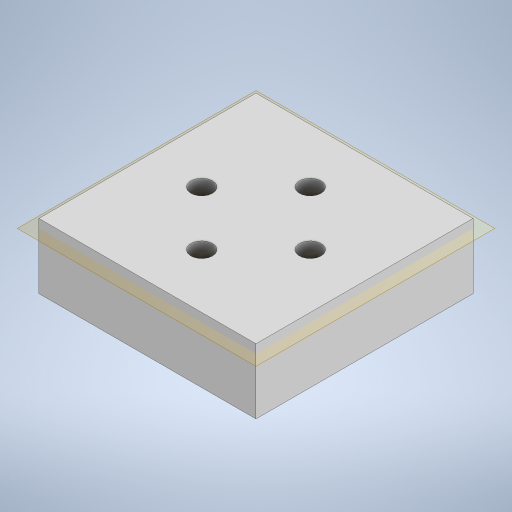
# Autodesk Inventor part: TestBauteil
Saved by Autodesk Inventor 2024.1 (Build 281209000, 209)
## iProperties
Created: 2023-11-30
Part Number: TestBauteil
Material: Generisch
Document SubType Name: Modeling
Designer: tobia
Density: 1 g/cm^3
Appearance: Vorgabe
Author: tobia
Autodesk Inventor part; units mm, degrees
ref_plane "YZ Plane" through (0, 0, 0) normal (1, 0, 0) x (0, 1, 0)
ref_plane "XZ Plane" through (0, 0, 0) normal (0, 1, 0) x (-1, 0, 0)
ref_plane "XY Plane" through (0, 0, 0) normal (0, 0, 1) x (1, 0, 0)
sketch "Skizze1" plane through (0, 0, 0) normal (0, 0, 1) x (1, 0, 0)
  line L0 (-25, 25) -> (25, 25)
  line L1 (25, 25) -> (25, -25)
  line L2 (25, -25) -> (-25, -25)
  line L3 (-25, -25) -> (-25, 25)
  point P0 (0, 0)
  point P1 (25, 0)
  point P2 (0, 25)
  dimension "d0" = 50
  dimension "d1" = 50
  constraints: 8 end point, 2 midpoint, 2 parallel, 1 horizontal, 1 horizontal alignment, 1 perpendicular, 1 vertical alignment
  measures "d0" distance of L0.end L1.end
  measures "d1" distance of L1.end L2.end
extrude "Extrusion1" add sketch "Skizze1" along normal blind 15
ref_plane "Arbeitsebene1" through (0, 0, 13) normal (0, 0, 1) x (1, 0, 0)
sketch "Skizze4" plane through (0, 0, 13) normal (0, 0, 1) x (1, 0, 0)
  circle A0 centre (-12.5, -12.5) radius 7.5
  line L0 (-25, 25) -> (-25, -25) projected
  circle A1 centre (12.5, -12.5) radius 7.5
  line L1 (25, -25) -> (25, 25) projected
  line L2 (-25, -25) -> (25, -25) projected
  circle A2 centre (-12.5, 12.5) radius 7.5
  line L3 (25, 25) -> (-25, 25) projected
  circle A3 centre (12.5, 12.5) radius 7.5
  point P0 (0, 0)
  dimension "d6" = 15
  dimension "d7" = 12.5
  dimension "d8" = 15
  dimension "d9" = 12.5
  dimension "d10" = 12.5
  dimension "d11" = 12.5
  dimension "d12" = 15
  dimension "d13" = 12.5
  dimension "d14" = 12.5
  dimension "d15" = 15
  constraints: 4 centre point
  measures "d6" diameter of A0
  measures "d7" distance from line of L0 A0.centre
  measures "d8" diameter of A1
  measures "d9" distance from line of L1 A1.centre
  measures "d10" distance from line of L2 A1.centre
  measures "d11" distance from line of L2 A0.centre
  measures "d12" diameter of A2
  measures "d13" distance from line of L0 A2.centre
  measures "d14" distance from line of L3 A2.centre
  measures "d15" diameter of A3
extrude "Extrusion2" cut sketch "Skizze4" against normal blind 8 contours A0 | A1 | A2 | A3
sketch "Skizze6" plane through (0, 0, 15) normal (0, 0, 1) x (1, 0, 0)
  circle A0 centre (-12.5, 0) radius 2.5
  circle A1 centre (0, 12.5) radius 2.5
  circle A2 centre (12.5, 0) radius 2.5
  circle A3 centre (0, -12.5) radius 2.5
  line L0 (25, 25) -> (-25, 25) projected
  line L1 (-25, 25) -> (-25, -25) projected
  line L2 (25, -25) -> (25, 25) projected
  point P0 (0, 0)
  dimension "d18" = 5
  dimension "d19" = 12.5
  dimension "d20" = 25
  dimension "d21" = 5
  dimension "d22" = 12.5
  dimension "d23" = 25
  dimension "d24" = 5
  dimension "d25" = 12.5
  dimension "d26" = 25
  dimension "d27" = 5
  dimension "d28" = 12.5
  dimension "d29" = 25
  constraints: 4 centre point
  measures "d18" diameter of A0
  measures "d19" distance of point (0, 0) A0.centre
  measures "d20" distance from line of L0 A0.centre
  measures "d21" diameter of A1
  measures "d22" distance of point (0, 0) A1.centre
  measures "d23" distance from line of L1 A1.centre
  measures "d24" diameter of A2
  measures "d25" distance of point (0, 0) A2.centre
  measures "d26" distance from line of A2.centre L0
  measures "d27" diameter of A3
  measures "d28" distance of point (0, 0) A3.centre
  measures "d29" distance from line of L2 A3.centre
extrude "Extrusion3" cut sketch "Skizze6" against normal blind 10
sketch "Skizze7" plane through (0, 0, 0) normal (0, 0, -1) x (-1, 0, 0)
  circle A0 centre (0, 12.5) radius 2.5 projected
  circle A1 centre (0, 12.5) radius 1
  circle A2 centre (0, -12.5) radius 2.5 projected
  circle A3 centre (0, -12.5) radius 1
  circle A4 centre (-12.5, 0) radius 2.5 projected
  circle A5 centre (-12.5, 0) radius 1
  circle A6 centre (12.5, 0) radius 2.5 projected
  circle A7 centre (12.5, 0) radius 1
  point P0 (0, 0)
  dimension "d32" = 2
  dimension "d33" = 2
  dimension "d34" = 2
  dimension "d35" = 2
  constraints: 4 centre point, 4 coincident
  measures "d32" diameter of A1
  measures "d33" diameter of A7
  measures "d34" diameter of A5
  measures "d35" diameter of A3
extrude "Extrusion4" cut sketch "Skizze7" against normal blind 10 contours A1 | A3 | A5 | A7
